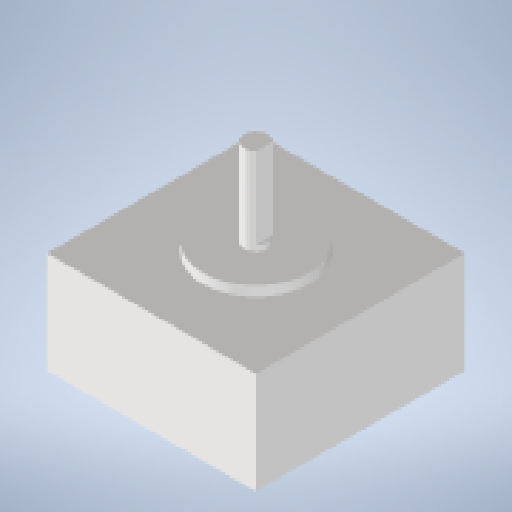
# Autodesk Inventor part: PancakeStepper
Saved by Autodesk Inventor 2023 (Build 270158000, 158)
## iProperties
Created: 2023-08-31
Part Number: PancakeStepper
Material: Steel, Carbon
Document SubType Name: Modeling
Designer: Felix
Density: 7.85 g/cm^3
Appearance: Semi-Polished
Author: Felix
Autodesk Inventor part; units mm, degrees
ref_plane "YZ Plane" through (0, 0, 0) normal (1, 0, 0) x (0, 1, 0)
ref_plane "XZ Plane" through (0, 0, 0) normal (0, 1, 0) x (-1, 0, 0)
ref_plane "XY Plane" through (0, 0, 0) normal (0, 0, 1) x (1, 0, 0)
sketch "Sketch1" plane through (0, 0, 0) normal (0, 1, 0) x (-1, 0, 0)
  line L0 (-21.5, 21.5) -> (21.5, 21.5)
  line L1 (21.5, 21.5) -> (21.5, -21.5)
  line L2 (21.5, -21.5) -> (-21.5, -21.5)
  line L3 (-21.5, -21.5) -> (-21.5, 21.5)
  line L4 (-21.5, 21.5) -> (21.5, -21.5) construction
  line L5 (21.5, 21.5) -> (-21.5, -21.5) construction
  point P0 (0, 0)
  dimension "d0" = 43
  dimension "d1" = 43
  constraints: 12 end point, 2 midpoint, 2 parallel, 1 horizontal, 1 perpendicular
  measures "d0" distance of L1.end L2.end
  measures "d1" distance of L0.end L1.end
extrude "Extrusion1" add sketch "Sketch1" along normal blind 21
sketch "Sketch2" plane through (0, 21, 0) normal (0, 1, 0) x (1, 0, 0)
  line L0 (21.5, 21.5) -> (-21.5, 21.5) construction
  line L1 (-21.5, 21.5) -> (-21.5, -21.5) construction
  line L2 (-21.5, -21.5) -> (21.5, -21.5) construction
  line L3 (21.5, -21.5) -> (21.5, 21.5) construction
  line L4 (21.5, -21.5) -> (-21.5, 21.5) construction
  line L5 (21.5, 21.5) -> (-21.5, -21.5) construction
  circle A0 centre (0, 0) radius 11
  dimension "d4" = 22
  constraints: 4 end point, 1 centre point, 1 coincident, 1 perpendicular, 1 point on line
  measures "d4" diameter of A0
extrude "Extrusion2" add sketch "Sketch2" along normal blind 2
sketch "Sketch3" plane through (0, 23, 0) normal (0, 1, 0) x (1, 0, 0)
  circle A0 centre (0, 0) radius 11 construction
  circle A1 centre (0, 0) radius 11 construction
  circle A2 centre (0, 0) radius 2.5
  dimension "d7" = 5
  constraints: 1 centre point, 1 coincident
  measures "d7" diameter of A2
extrude "Extrusion3" add sketch "Sketch3" along normal blind 18
sketch "Sketch4" plane through (0, 41, 0) normal (0, 1, 0) x (1, 0, 0)
  circle A0 centre (0, 0) radius 2.5 projected
  line L0 (1.7854, 1.75) -> (1.7854, -1.75)
  dimension "d11" = 3.5
  constraints: 2 end point, 2 point on circle, 1 vertical
  measures "d11" distance of L0.start L0.end
extrude "Extrusion4" cut sketch "Sketch4" against normal blind 16.75 contours A0 L0 picked at (1.8866, -0.4578)
chamfer "Chamfer1" distance 4.0426 angle 45 4 edges at (-21.5, 10.5, 21.5) (21.5, 10.5, 21.5) (21.5, 10.5, -21.5) (-21.5, 10.5, -21.5)
sketch "Sketch5" plane through (0, 21, 0) normal (0, 1, 0) x (1, 0, 0)
  line L0 (-21.5, 17.4574) -> (-17.4574, 21.5) construction
  line L1 (-21.5, 17.4574) -> (-21.5, -17.4574) construction
  line L2 (-17.4574, -21.5) -> (-21.5, -17.4574) construction
  line L3 (-17.4574, -21.5) -> (17.4574, -21.5) construction
  line L4 (21.5, -17.4574) -> (17.4574, -21.5) construction
  line L5 (21.5, -17.4574) -> (21.5, 17.4574) construction
  line L6 (17.4574, 21.5) -> (21.5, 17.4574) construction
  line L7 (17.4574, 21.5) -> (-17.4574, 21.5) construction
  circle A0 centre (0, 0) radius 11 construction
  line L8 (15.5, -15.5) -> (-15.5, -15.5) construction
  line L9 (-15.5, -15.5) -> (-15.5, 15.5) construction
  line L10 (-15.5, 15.5) -> (15.5, 15.5) construction
  line L11 (15.5, 15.5) -> (15.5, -15.5) construction
  circle A1 centre (0, 0) radius 2.5 construction
  line L12 (15.5, -15.5) -> (-15.5, 15.5) construction
  line L13 (-15.5, -15.5) -> (15.5, 15.5) construction
  dimension "d17" = 31
  dimension "d18" = 31
  constraints: 12 end point, 4 coincident, 2 midpoint, 2 parallel, 1 horizontal, 1 perpendicular
  measures "d17" distance of L9.end L10.end
  measures "d18" distance of L8.end L9.end
hole "Hole1" at (-15.5, 21, 15.5) at (-15.5, 21, -15.5) at (15.5, 21, -15.5) at (15.5, 21, 15.5) direction (0, -1, 0) diameter 2.459 depth 3.5 thread size "M3x0.5" class "6H" standard "ISO Metric profile"
body "Solid1"
